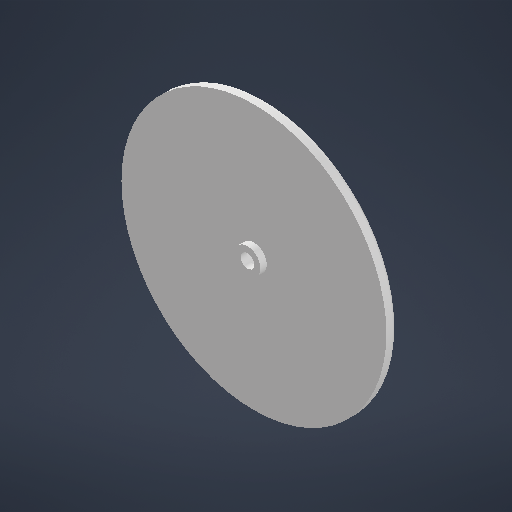
# Autodesk Inventor part: center_disk
Saved by Autodesk Inventor 2026 (Build 300175050, 175E)
## iProperties
Created: 2026-05-09
Part Number: center_disk
Material: Generic
Document SubType Name: Modeling
Designer: sniel
Density: 1 g/cm^3
Appearance: Default
Author: sniel
Autodesk Inventor part; units mm, degrees
ref_plane "YZ Plane" through (0, 0, 0) normal (1, 0, 0) x (0, 1, 0)
ref_plane "XZ Plane" through (0, 0, 0) normal (0, 1, 0) x (-1, 0, 0)
ref_plane "XY Plane" through (0, 0, 0) normal (0, 0, 1) x (1, 0, 0)
sketch "Sketch1" plane through (0, 0, 0) normal (0, 0, 1) x (1, 0, 0)
  arc A0 (-1.9795, 6.7143) -> (1.9795, 6.7143) centre (0, 7) ccw
  arc A1 (-1.9795, 6.7143) -> (-1.9795, -6.7143) centre (0, 0) ccw
  arc A2 (1.9795, -6.7143) -> (-1.9795, -6.7143) centre (0, -7) ccw
  arc A3 (1.9795, -6.7143) -> (1.9795, 6.7143) centre (0, 0) ccw
  line L0 (3.6, 1.9621) -> (3.6, -1.9621)
  arc A4 (3.6, 1.9621) -> (3.6, -1.9621) centre (0, 0) ccw
  circle A5 centre (0, -7) radius 1.75
  circle A6 centre (0, 7) radius 1.75
  circle A7 centre (0, 0) radius 7.5
  circle A8 centre (0, 0) radius 102.5
  point P0 (0, 0)
  point P1 (-1.7242, 7.2991)
  point P2 (1.7242, 7.2991)
  point P3 (1.7242, -7.2991)
  point P4 (-1.7242, -7.2991)
  dimension "d0" = 3.5
  dimension "d1" = 3.5
  dimension "d2" = 15
  dimension "d3" = 205
  constraints: 10 point on circle, 9 centre point, 4 coincident, 2 end point
  measures "d0" diameter of A5
  measures "d1" diameter of A6
  measures "d2" diameter of A7
  measures "d3" diameter of A8
extrude "Extrusion1" add sketch "Sketch1" against normal blind 8.25 contours A5 A7 | A7 A5 | A7 A6 | A6 A7 | A8
fillet "Fillet1" radius 3.5 1 edges at (-102.5, 0, -8.25)
sketch "Sketch2" plane through (0, 0, 0) normal (0, 0, 1) x (1, 0, 0)
  circle A0 centre (0, 0) radius 5.25
  arc A1 (1.7242, -7.2991) -> (-1.7242, -7.2991) centre (0, -7) ccw projected
  circle A2 centre (0, 0) radius 10
  dimension "d7" = 20
  constraints: 2 centre point, 2 coincident, 1 tangent
  measures "d7" diameter of A2
extrude "Extrusion2" add sketch "Sketch2" along normal blind 5
body "Solid1"
